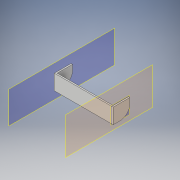
# Autodesk Inventor part: Top Basic layout
Saved by Autodesk Inventor 2018 (Build 220112000, 112)
## iProperties
Created: 2018-01-18
Part Number: Top Basic layout
Material: Generic
Document SubType Name: Modeling
Designer: mwood
Density: 1 g/cm^3
Appearance: Default
Author: mwood
Autodesk Inventor part; units mm, degrees
ref_plane "YZ Plane" through (0, 0, 0) normal (1, 0, 0) x (0, 1, 0)
ref_plane "XZ Plane" through (0, 0, 0) normal (0, 1, 0) x (-1, 0, 0)
ref_plane "XY Plane" through (0, 0, 0) normal (0, 0, 1) x (1, 0, 0)
sketch "Sketch1" plane through (0, 0, 0) normal (0, 0, 1) x (1, 0, 0)
  line L0 (-131.0833, 65.4113) -> (124.5042, 65.4113)
  line L1 (124.5042, 65.4113) -> (124.5042, -0.7128)
  line L2 (124.5042, -0.7128) -> (-131.0833, -0.7128)
  line L3 (-131.0833, -0.7128) -> (-131.0833, 65.4113)
  point P0 (0, 0)
  constraints: 8 end point, 2 parallel, 1 horizontal, 1 perpendicular
extrude "Extrusion1" add sketch "Sketch1" along normal blind 6.35
ref_plane "Work Plane2" through (124.5042, 65.4113, 3.175) normal (1, 0, 0) x (0, 0, -1)
sketch "Sketch4" plane through (124.5042, 65.4113, 3.175) normal (1, 0, 0) x (0, 0, -1)
  line L0 (3.175, -66.1241) -> (3.175, 0) projected
  line L1 (3.175, -66.1241) -> (69.85, -66.1241)
  line L2 (69.85, -66.1241) -> (69.85, 0)
  line L3 (69.85, 0) -> (3.175, 0)
  line L4 (3.175, 0) -> (3.175, -66.1241)
  point P0 (3.175, -65.4113)
  dimension "d2" = 66.1241
  dimension "d3" = 66.675
  constraints: 8 end point, 2 parallel, 1 horizontal, 1 perpendicular
  measures "d2" distance of L1.end L2.end
  measures "d3" distance of L2.end L3.end
extrude "Extrusion2" add sketch "Sketch4" against normal blind 6.35
fillet "Fillet1" radius 44.45 1 edges at (121.3292, -0.7128, -66.675)
ref_plane "Work Plane3" through (-131.0833, -0.7128, 0) normal (-1, 0, 0) x (0, 0, 1)
sketch "Sketch5" plane through (-131.0833, -0.7128, 0) normal (-1, 0, 0) x (0, 0, 1)
  line L0 (0, 66.1241) -> (-66.675, 66.1241) projected
  line L1 (0, 66.1241) -> (-66.675, 66.1241)
  line L2 (-66.675, 66.1241) -> (-66.675, 0)
  line L3 (-66.675, 0) -> (0, 0)
  line L4 (0, 0) -> (0, 66.1241)
  point P0 (0, 0.7128)
  constraints: 8 end point, 2 parallel, 1 horizontal, 1 perpendicular
extrude "Extrusion3" add sketch "Sketch5" against normal blind 6.35
fillet "Fillet2" radius 44.45 1 edges at (-127.9083, -0.7128, -66.675)
ref_plane "Work Plane4" through (118.1542, 65.4113, -66.675) normal (-1, 0, 0) x (0, 0, 1)
sketch "Sketch6" plane through (118.1542, 65.4113, -66.675) normal (-1, 0, 0) x (0, 0, 1)
  circle A0 centre (60.325, -12.7) radius 1.5875
  point P0 (66.675, -65.4113)
  dimension "d11" = 3.175
  constraints: 1 centre point
  measures "d11" diameter of A0
extrude "Extrusion4" add sketch "Sketch6" along normal blind 5.08
body "Solid1"
